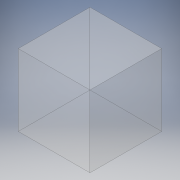
# Autodesk Inventor part: Cube
Saved by Autodesk Inventor 2019 (Build 230136000, 136)
## iProperties
Created: 2019-09-28
Part Number: Cube
Material: Generic
Document SubType Name: Modeling
Designer: james
Density: 1 g/cm^3
Appearance: Polycarbonate - Clear
Author: james
Autodesk Inventor part; units mm, degrees
ref_plane "YZ Plane" through (0, 0, 0) normal (1, 0, 0) x (0, 1, 0)
ref_plane "XZ Plane" through (0, 0, 0) normal (0, 1, 0) x (-1, 0, 0)
ref_plane "XY Plane" through (0, 0, 0) normal (0, 0, 1) x (1, 0, 0)
sketch "Sketch1" plane through (0, 0, 0) normal (0, 1, 0) x (-1, 0, 0)
  line L0 (254.1468, 464.6879) -> (-203.0532, 464.6879)
  line L1 (-203.0532, 464.6879) -> (-203.0532, 7.4879)
  line L2 (-203.0532, 7.4879) -> (254.1468, 7.4879)
  line L3 (254.1468, 7.4879) -> (254.1468, 464.6879)
  point P0 (0, 0)
  dimension "d0" = 457.2
  dimension "d1" = 457.2
  constraints: 8 end point, 2 parallel, 1 horizontal, 1 perpendicular
  measures "d0" distance of L0.start L0.end
  measures "d1" distance of L2.end L0.start
extrude "Extrusion1" add sketch "Sketch1" along normal blind 457.2
body "Solid1"
